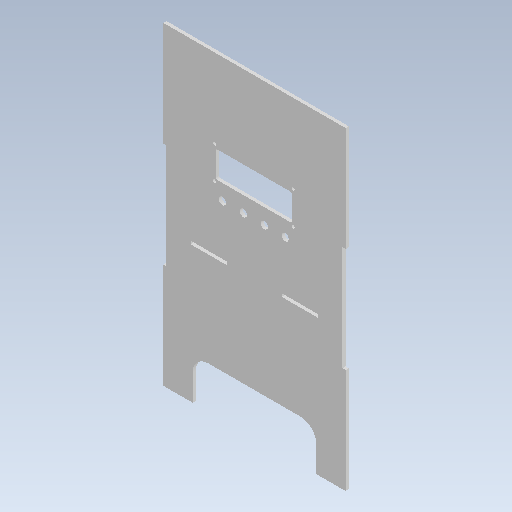
# Autodesk Inventor part: Pared_Lateral
Saved by Autodesk Inventor 2020.1 (Build 241239000, 239)
## iProperties
Created: 2019-12-08
Part Number: Pared_Lateral
Material: Generic
Document SubType Name: Modeling
Designer: Daniel
Density: 1 g/cm^3
Appearance: Default
Author: Daniel
Autodesk Inventor part; units mm, degrees
ref_plane "YZ Plane" through (0, 0, 0) normal (1, 0, 0) x (0, 1, 0)
ref_plane "XZ Plane" through (0, 0, 0) normal (0, 1, 0) x (-1, 0, 0)
ref_plane "XY Plane" through (0, 0, 0) normal (0, 0, 1) x (1, 0, 0)
sketch "Sketch1" plane through (0, 0, 0) normal (0, 0, 1) x (1, 0, 0)
  line L0 (-84, -131.5) -> (84, -131.5)
  line L1 (84, -131.5) -> (84, 168.5)
  line L2 (84, 168.5) -> (-84, 168.5)
  line L3 (-84, 168.5) -> (-84, -131.5)
  line L4 (-84, 1.5) -> (-84, -1.5) projected
  line L5 (84, -1.5) -> (84, 1.5) projected
  line L6 (61, -1.5) -> (84, -1.5) projected
  line L7 (26, -1.5) -> (61, -1.5) projected
  line L8 (61, 1.5) -> (61, -1.5) projected
  line L9 (26, 1.5) -> (61, 1.5) projected
  line L10 (26, 1.5) -> (26, -1.5) projected
  point P0 (0, 0)
  dimension "d0" = 300
  dimension "d1" = 170
  constraints: 8 end point, 2 collinear, 2 parallel, 1 horizontal, 1 perpendicular
  measures "d0" distance of L0.end L1.end
  measures "d1" distance between parallel lines of L2 L6
extrude "Extrusion1" add sketch "Sketch1" along normal blind 3
sketch "Sketch2" plane through (0, 0, 0) normal (0, 0, -1) x (-1, 0, 0)
  line L0 (84, 1.5) -> (84, -1.5)
  line L1 (84, -1.5) -> (61, -1.5)
  line L2 (61, 1.5) -> (61, -1.5)
  line L3 (26, 1.5) -> (61, 1.5)
  line L4 (26, -1.5) -> (26, 1.5)
  line L5 (26, -1.5) -> (-26, -1.5)
  line L6 (-26, 1.5) -> (-26, -1.5)
  line L7 (-61, 1.5) -> (-26, 1.5)
  line L8 (-61, -1.5) -> (-61, 1.5)
  line L9 (-61, -1.5) -> (-84, -1.5)
  line L10 (-84, -1.5) -> (-84, 1.5)
  line L11 (-84, 1.5) -> (-61, 1.5)
  line L12 (61, 1.5) -> (84, 1.5)
  line L13 (61, -1.5) -> (26, -1.5)
  line L14 (-26, 1.5) -> (26, 1.5)
  line L15 (-26, -1.5) -> (-61, -1.5)
  point P0 (0, 0)
  constraints: 32 end point, 10 horizontal, 6 vertical, 12 other
extrude "Extrusion2" cut sketch "Sketch2" against normal blind 10 contours L2 L13 L4 L3
sketch "Sketch3" plane through (0, 0, 3) normal (0, 0, 1) x (1, 0, 0)
  line L0 (84, -131.5) -> (84, 168.5) projected
  line L1 (84, -131.5) -> (87, -131.5)
  line L2 (87, -131.5) -> (87, -31.5)
  line L3 (87, -31.5) -> (84, -31.5)
  line L4 (84, -31.5) -> (84, -131.5)
  line L5 (-61, -1.5) -> (-26, -1.5) projected
  line L6 (-26, -1.5) -> (-26, 1.5) projected
  line L7 (-26, 1.5) -> (-61, 1.5) projected
  line L8 (-61, 1.5) -> (-61, -1.5) projected
  line L9 (26, 1.5) -> (26, -1.5) projected
  line L10 (26, -1.5) -> (61, -1.5) projected
  line L11 (61, -1.5) -> (61, 1.5) projected
  line L12 (61, 1.5) -> (26, 1.5) projected
  line L13 (-84, 168.5) -> (84, 168.5) projected
  line L14 (84, 168.5) -> (84, -131.5) projected
  line L15 (84, -131.5) -> (-84, -131.5) projected
  line L16 (-84, -131.5) -> (-84, 168.5) projected
  line L17 (87, 168.5) -> (84, 168.5)
  line L18 (84, 68.5) -> (87, 68.5)
  line L19 (87, 68.5) -> (87, 168.5)
  line L20 (84, 168.5) -> (84, 68.5)
  line L21 (-84, -31.5) -> (-87, -31.5)
  line L22 (-87, -131.5) -> (-84, -131.5)
  line L23 (-84, -131.5) -> (-84, -31.5)
  line L24 (-87, -31.5) -> (-87, -131.5)
  line L25 (-84, 168.5) -> (-87, 168.5)
  line L26 (-87, 68.5) -> (-84, 68.5)
  line L27 (-84, 68.5) -> (-84, 168.5)
  line L28 (-87, 168.5) -> (-87, 68.5)
  point P0 (0, 0)
  dimension "d6" = 100
  dimension "d7" = 3
  dimension "d10" = 200
  dimension "d13" = 171
  constraints: 32 end point, 2 horizontal, 2 parallel, 1 perpendicular, 1 vertical, 24 other
  measures "d6" distance of L1.end L2.end
  measures "d7" distance of L0.start L1.end
  measures "d10" distance of L3.end L17.end
  measures "d13" distance of L3.end L21.end
extrude "Extrusion3" add sketch "Sketch3" against normal up to surface (3 mm away) contours L0 L3 L2 L1 | L22 L24 L21 L16 | L0 L17 L19 L18 | L26 L28 L25 L16
sketch "Sketch4" plane through (0, 0, 3) normal (0, 0, 1) x (1, 0, 0)
  line L0 (-59, -131.5) -> (59, -131.5)
  line L1 (59, -131.5) -> (59, -91.5)
  line L2 (59, -91.5) -> (-59, -91.5)
  line L3 (-59, -91.5) -> (-59, -131.5)
  line L4 (-87, -131.5) -> (87, -131.5) projected
  line L5 (87, -131.5) -> (87, -31.5) projected
  line L6 (-87, -31.5) -> (-87, -131.5) projected
  point P0 (0, 0)
  dimension "d18" = 28
  dimension "d19" = 28
  dimension "d20" = 40
  constraints: 8 end point, 2 parallel, 1 collinear, 1 horizontal, 1 perpendicular
  measures "d18" distance between parallel lines of L5 L1
  measures "d19" distance between parallel lines of L6 L3
  measures "d20" distance of L0.end L1.end
extrude "Extrusion4" cut sketch "Sketch4" against normal blind 10
fillet "Fillet1" radius 15 2 edges at (59, -91.5, 1.5) (-59, -91.5, 1.5)
sketch "Sketch5" plane through (0, 0, 0) normal (0, 0, -1) x (-1, 0, 0)
  circle A0 centre (-29.3933, 49.5) radius 3.5
  circle A1 centre (-9.3933, 49.5) radius 3.5
  circle A2 centre (10.6067, 49.5) radius 3.5
  circle A3 centre (30.6067, 49.5) radius 3.5
  line L0 (-34.0433, 89.15) -> (35.2567, 89.15)
  arc A4 (36.2567, 88.15) -> (35.2567, 89.15) centre (35.2567, 88.15) ccw
  line L1 (36.2567, 88.15) -> (36.2567, 65.85)
  arc A5 (35.2567, 64.85) -> (36.2567, 65.85) centre (35.2567, 65.85) ccw
  line L2 (35.2567, 64.85) -> (-34.0433, 64.85)
  arc A6 (-35.0433, 65.85) -> (-34.0433, 64.85) centre (-34.0433, 65.85) ccw
  line L3 (-35.0433, 65.85) -> (-35.0433, 88.15)
  arc A7 (-34.0433, 89.15) -> (-35.0433, 88.15) centre (-34.0433, 88.15) ccw
  line L4 (-34.5433, 88.15) -> (-34.5433, 65.85)
  arc A8 (-34.5433, 65.85) -> (-34.0433, 65.35) centre (-34.0433, 65.85) ccw
  line L5 (-34.0433, 65.35) -> (35.2567, 65.35)
  arc A9 (35.2567, 65.35) -> (35.7567, 65.85) centre (35.2567, 65.85) ccw
  line L6 (35.7567, 65.85) -> (35.7567, 88.15)
  arc A10 (35.7567, 88.15) -> (35.2567, 88.65) centre (35.2567, 88.15) ccw
  line L7 (35.2567, 88.65) -> (33.3925, 88.65)
  spline S0 degree 3 poles (33.3925, 88.65) (33.3126, 88.65) (33.217, 88.642) (32.9717, 88.6132) (32.7737, 88.5819) (32.6067, 88.5819) knots 0 0 0 0 0.32369 0.32369 1 1 1 1
  line L8 (32.6067, 88.5819) -> (-31.3933, 88.5819)
  spline S1 degree 3 poles (-31.3933, 88.5819) (-31.5603, 88.5819) (-31.7583, 88.6132) (-32.0036, 88.642) (-32.0992, 88.65) (-32.1791, 88.65) knots 0 0 0 0 0.67631 0.67631 1 1 1 1
  line L9 (-32.1791, 88.65) -> (-34.0433, 88.65)
  arc A11 (-34.0433, 88.65) -> (-34.5433, 88.15) centre (-34.0433, 88.15) ccw
  line L10 (-33.3933, 69) -> (-33.3933, 86)
  line L11 (-33.3933, 86) -> (34.6067, 86)
  line L12 (34.6067, 86) -> (34.6067, 69)
  line L13 (34.6067, 69) -> (-33.3933, 69)
  circle A12 centre (38.1067, 93) radius 1.5
  circle A13 centre (-36.8933, 93) radius 1.5
  circle A14 centre (-36.8933, 62) radius 1.5
  circle A15 centre (38.1067, 62) radius 1.5
  line L14 (36.7567, 65.85) -> (36.7567, 88.15)
  arc A16 (36.7567, 88.15) -> (35.2567, 89.65) centre (35.2567, 88.15) ccw
  line L15 (35.2567, 89.65) -> (-34.0433, 89.65)
  arc A17 (-34.0433, 89.65) -> (-35.5433, 88.15) centre (-34.0433, 88.15) ccw
  line L16 (-35.5433, 88.15) -> (-35.5433, 65.85)
  arc A18 (-35.5433, 65.85) -> (-34.0433, 64.35) centre (-34.0433, 65.85) ccw
  line L17 (-34.0433, 64.35) -> (35.2567, 64.35)
  arc A19 (35.2567, 64.35) -> (36.7567, 65.85) centre (35.2567, 65.85) ccw
  point P0 (0, 0)
  dimension "d24" = 0.5
  constraints: 36 end point, 24 point on circle, 16 centre point, 8 horizontal, 6 vertical, 61 other
  measures "d24" distance between parallel lines of L1 L14
extrude "Extrusion5" cut sketch "Sketch5" against normal blind 10 contours A0 | A1 | A2 | A3 | L0 A4 L1 A5 L2 A6 L3 A7 | A11 L9 S1 L8 S0 L7 A10 L6 A9 L5 A8 L4 | L10 L11 L12 L13 | A12 | A13 | A14 | A15 | A19 L17 A18 L16 A17 L15 A16 L14
body "Solid1"
